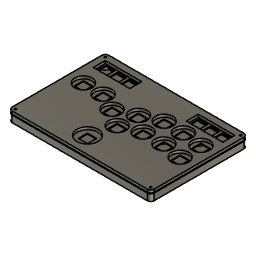
PitBox (Autodesk Fusion 360 design; units mm, degrees)
Autodesk Fusion 360 part; units mm, degrees
sketch "Sketch2" plane through (0, 0, 0) normal (0, 0, 1) x (1, 0, 0)
  circle A0 centre (22.2936, -55.3178) radius 12.0327
  circle A1 centre (51.9241, -55.2175) radius 12.0327
  circle A2 centre (78.346, -68.2028) radius 12.0327
  circle A3 centre (106.2419, -56.2403) radius 12.0327
  circle A4 centre (133.2453, -44.4382) radius 12.0327
  circle A5 centre (162.9862, -45.1702) radius 12.0327
  circle A6 centre (192.5566, -48.2686) radius 12.0327
  circle A7 centre (103.5847, -85.6403) radius 12.0327
  circle A8 centre (131.5808, -74.52) radius 12.0327
  circle A9 centre (162.7756, -74.3195) radius 12.0327
  circle A10 centre (192.2758, -79.3532) radius 12.0327
  circle A11 centre (93.8883, -120.7958) radius 15.0409
  line L0 (15.3935, -48.4178) -> (29.1935, -48.4178)
  line L1 (29.1935, -48.4178) -> (29.1935, -62.2178)
  line L2 (29.1935, -62.2178) -> (15.3935, -62.2178)
  line L3 (15.3935, -62.2178) -> (15.3935, -48.4178)
  line L4 (45.0241, -48.3175) -> (58.8241, -48.3175)
  line L5 (58.8241, -48.3175) -> (58.8241, -62.1175)
  line L6 (58.8241, -62.1175) -> (45.0241, -62.1175)
  line L7 (45.0241, -62.1175) -> (45.0241, -48.3175)
  line L8 (71.446, -61.3028) -> (85.246, -61.3028)
  line L9 (85.246, -61.3028) -> (85.246, -75.1028)
  line L10 (85.246, -75.1028) -> (71.446, -75.1028)
  line L11 (71.446, -75.1028) -> (71.446, -61.3028)
  line L12 (99.3419, -49.3403) -> (113.1419, -49.3403)
  line L13 (113.1419, -49.3403) -> (113.1419, -63.1403)
  line L14 (113.1419, -63.1403) -> (99.3419, -63.1403)
  line L15 (99.3419, -63.1403) -> (99.3419, -49.3403)
  line L16 (126.3453, -37.5382) -> (140.1453, -37.5382)
  line L17 (140.1453, -37.5382) -> (140.1453, -51.3382)
  line L18 (140.1453, -51.3382) -> (126.3453, -51.3382)
  line L19 (126.3453, -51.3382) -> (126.3453, -37.5382)
  line L20 (156.0862, -38.2702) -> (169.8862, -38.2702)
  line L21 (169.8862, -38.2702) -> (169.8862, -52.0702)
  line L22 (169.8862, -52.0702) -> (156.0862, -52.0702)
  line L23 (156.0862, -52.0702) -> (156.0862, -38.2702)
  line L24 (185.6566, -41.3686) -> (199.4566, -41.3686)
  line L25 (199.4566, -41.3686) -> (199.4566, -55.1686)
  line L26 (199.4566, -55.1686) -> (185.6566, -55.1686)
  line L27 (185.6566, -55.1686) -> (185.6566, -41.3686)
  line L28 (185.3758, -72.4532) -> (199.1758, -72.4532)
  line L29 (199.1758, -72.4532) -> (199.1758, -86.2532)
  line L30 (199.1758, -86.2532) -> (185.3758, -86.2532)
  line L31 (185.3758, -86.2532) -> (185.3758, -72.4532)
  line L32 (155.8756, -67.4195) -> (169.6756, -67.4195)
  line L33 (169.6756, -67.4195) -> (169.6756, -81.2195)
  line L34 (169.6756, -81.2195) -> (155.8756, -81.2195)
  line L35 (155.8756, -81.2195) -> (155.8756, -67.4195)
  line L36 (124.6808, -67.62) -> (138.4808, -67.62)
  line L37 (138.4808, -67.62) -> (138.4808, -81.42)
  line L38 (138.4808, -81.42) -> (124.6808, -81.42)
  line L39 (124.6808, -81.42) -> (124.6808, -67.62)
  line L40 (96.6847, -78.7403) -> (110.4846, -78.7403)
  line L41 (110.4846, -78.7403) -> (110.4846, -92.5403)
  line L42 (110.4846, -92.5403) -> (96.6847, -92.5403)
  line L43 (96.6847, -92.5403) -> (96.6847, -78.7403)
  line L44 (86.9883, -113.8959) -> (100.7883, -113.8959)
  line L45 (100.7883, -113.8959) -> (100.7883, -127.6959)
  line L46 (100.7883, -127.6959) -> (86.9883, -127.6959)
  line L47 (86.9883, -127.6959) -> (86.9883, -113.8959)
  line L48 (12.2471, -11.7471) -> (26.0471, -11.7471)
  line L49 (26.0471, -11.7471) -> (26.0471, -25.5471)
  line L50 (26.0471, -25.5471) -> (12.2471, -25.5471)
  line L51 (12.2471, -25.5471) -> (12.2471, -11.7471)
  line L52 (30.2471, -11.7471) -> (44.0471, -11.7471)
  line L53 (44.0471, -11.7471) -> (44.0471, -25.5471)
  line L54 (44.0471, -25.5471) -> (30.2471, -25.5471)
  line L55 (30.2471, -25.5471) -> (30.2471, -11.7471)
  line L56 (48.2471, -11.7471) -> (62.0471, -11.7471)
  line L57 (62.0471, -11.7471) -> (62.0471, -25.5471)
  line L58 (62.0471, -25.5471) -> (48.2471, -25.5471)
  line L59 (48.2471, -25.5471) -> (48.2471, -11.7471)
  line L60 (152.5223, -11.7471) -> (166.3223, -11.7471)
  line L61 (166.3223, -11.7471) -> (166.3223, -25.5471)
  line L62 (166.3223, -25.5471) -> (152.5223, -25.5471)
  line L63 (152.5223, -25.5471) -> (152.5223, -11.7471)
  line L64 (170.5223, -11.7471) -> (184.3223, -11.7471)
  line L65 (184.3223, -11.7471) -> (184.3223, -25.5471)
  line L66 (184.3223, -25.5471) -> (170.5223, -25.5471)
  line L67 (170.5223, -25.5471) -> (170.5223, -11.7471)
  line L68 (188.5223, -11.7471) -> (202.3223, -11.7471)
  line L69 (202.3223, -11.7471) -> (202.3223, -25.5471)
  line L70 (202.3223, -25.5471) -> (188.5223, -25.5471)
  line L71 (188.5223, -25.5471) -> (188.5223, -11.7471)
  line L72 (67.846, -4.145) -> (88.846, -4.145)
  line L73 (88.846, -4.145) -> (88.846, -55.145)
  line L74 (88.846, -55.145) -> (67.846, -55.145)
  line L75 (67.846, -55.145) -> (67.846, -4.145)
  line L76 (74.346, -2.845) -> (82.346, -2.845)
  line L77 (82.346, -2.845) -> (82.346, -4.145)
  line L78 (82.346, -4.145) -> (74.346, -4.145)
  line L79 (74.346, -4.145) -> (74.346, -2.845)
  circle A12 centre (72.646, -52.745) radius 1.25
  circle A13 centre (83.9813, -52.745) radius 1.25
  circle A14 centre (84.046, -6.145) radius 1.25
  circle A15 centre (72.646, -6.145) radius 1.25
  line L80 (0.0725, -0.0725) -> (214.4223, -0.0725)
  line L81 (214.4223, -0.0725) -> (214.4223, -145.9094)
  line L82 (214.4223, -145.9094) -> (0.0725, -145.9094)
  line L83 (0.0725, -145.9094) -> (0.0725, -0.0725)
  line L84 (10.1471, -10.1471) -> (64.1471, -10.1471)
  line L85 (64.1471, -10.1471) -> (64.1471, -27.1471)
  line L86 (64.1471, -27.1471) -> (10.1471, -27.1471)
  line L87 (10.1471, -27.1471) -> (10.1471, -10.1471)
  line L88 (150.4223, -10.1471) -> (204.4223, -10.1471)
  line L89 (204.4223, -10.1471) -> (204.4223, -27.1471)
  line L90 (204.4223, -27.1471) -> (150.4223, -27.1471)
  line L91 (150.4223, -27.1471) -> (150.4223, -10.1471)
  circle A16 centre (5.0725, -5.0725) radius 1.5
  circle A17 centre (209.4223, -5.0725) radius 1.5
  circle A18 centre (5.0725, -140.9094) radius 1.5
  circle A19 centre (209.4223, -140.9094) radius 1.5
  circle A20 centre (22.2936, -55.3178) radius 13.0327
  circle A21 centre (51.9241, -55.2175) radius 13.0327
  circle A22 centre (78.346, -68.2028) radius 13.0327
  circle A23 centre (106.2419, -56.2403) radius 13.0327
  circle A24 centre (133.2453, -44.4382) radius 13.0327
  circle A25 centre (162.9862, -45.1702) radius 13.0327
  circle A26 centre (192.5566, -48.2686) radius 13.0327
  circle A27 centre (103.5847, -85.6403) radius 13.0327
  circle A28 centre (131.5808, -74.52) radius 13.0327
  circle A29 centre (162.7756, -74.3195) radius 13.0327
  circle A30 centre (192.2758, -79.3532) radius 13.0327
  circle A31 centre (93.8883, -120.7958) radius 16.0409
  circle A32 centre (72.646, -6.145) radius 1
  circle A33 centre (84.046, -6.145) radius 1
  circle A34 centre (72.646, -6.145) radius 2
  circle A35 centre (84.046, -6.145) radius 2
  circle A36 centre (72.646, -52.745) radius 1
  circle A37 centre (83.9813, -52.745) radius 1
  circle A38 centre (72.646, -52.745) radius 2
  circle A39 centre (83.9813, -52.745) radius 2
  line L92 (72.646, -6.145) -> (84.046, -6.145)
  line L93 (84.846, 0.355) -> (71.846, 0.355)
  line L94 (71.846, 0.355) -> (71.846, -12.645)
  line L95 (71.846, -12.645) -> (84.846, -12.645)
  line L96 (84.846, -12.645) -> (84.846, 0.355)
  line L97 (84.846, 0.355) -> (71.846, -12.645) construction
  line L98 (71.846, 0.355) -> (84.846, -12.645) construction
  point P0 (34.3263, -55.3178)
  point P1 (63.9569, -55.2175)
  point P2 (90.3787, -68.2028)
  point P3 (118.2746, -56.2403)
  point P4 (145.2781, -44.4382)
  point P5 (175.019, -45.1702)
  point P6 (204.5894, -48.2686)
  point P7 (115.6174, -85.6403)
  point P8 (143.6135, -74.52)
  point P9 (174.8084, -74.3195)
  point P10 (204.3086, -79.3532)
  point P11 (108.9292, -120.7958)
  point P12 (73.896, -52.745)
  point P13 (85.2313, -52.745)
  point P14 (85.296, -6.145)
  point P15 (73.896, -6.145)
  point P16 (78.346, -6.145)
  dimension "d36" = 3
  dimension "d37" = 3
  dimension "d38" = 3
  dimension "d39" = 3
  dimension "d40" = 5
  dimension "d41" = 5
  dimension "d42" = 5
  dimension "d43" = 5
  dimension "d44" = 5
  dimension "d45" = 5
  dimension "d46" = 5
  dimension "d47" = 5
  dimension "d48" = -1
  dimension "d49" = -1
  dimension "d50" = -1
  dimension "d51" = -1
  dimension "d52" = -1
  dimension "d53" = -1
  dimension "d54" = -1
  dimension "d55" = -1
  dimension "d56" = -1
  dimension "d57" = -1
  dimension "d58" = -1
  dimension "d59" = -1
  dimension "d64" = 2
  dimension "d65" = 2
  dimension "d66" = 4
  dimension "d67" = 4
  dimension "d68" = 2
  dimension "d69" = 2
  dimension "d70" = 4
  dimension "d71" = 4
  dimension "d85" = 13
  dimension "d86" = 13
  constraint concentric A15 A32
  constraint concentric A14 A33
  constraint concentric A15 A34
  constraint concentric A33 A35
  constraint concentric A12 A36
  constraint concentric A13 A37
  constraint concentric A12 A38
  constraint concentric A37 A39
  constraint coincident A15.centre A32.centre
  constraint coincident A14.centre A33.centre
  constraint horizontal L93
  constraint perpendicular L93 L94
  constraint parallel L93 L95
  constraint parallel L94 L96
  constraint coincident L97 P16
  constraint coincident L98 P16
  constraint midpoint L92 P16
  measures "d36" diameter of A16
  measures "d37" diameter of A17
  measures "d38" diameter of A18
  measures "d39" diameter of A19
  measures "d40" distance of L80 A16.centre
  measures "d41" distance of L83 A16.centre
  measures "d42" distance of L80 A17.centre
  measures "d43" distance of L81 A17.centre
  measures "d44" distance of L81 A19.centre
  measures "d45" distance of L82 A19.centre
  measures "d46" distance of L82 A18.centre
  measures "d47" distance of L83 A18.centre
  measures "d64" diameter of A32
  measures "d65" diameter of A33
  measures "d66" diameter of A34
  measures "d67" diameter of A35
  measures "d68" diameter of A36
  measures "d69" diameter of A37
  measures "d70" diameter of A38
  measures "d71" diameter of A39
  measures "d85" distance of L94.end L95.end
  measures "d86" distance of L93.end L94.end
extrude "Extrude1" add sketch "Sketch2" along normal blind 4 contours L72 L76 L77 L78 L79 | L72 L78 A34 A35 L92 | L72 L76 L77 L79 L80 L94 L96 | L72 A34 L94 | A15 A34 L92 L94 | L72 A35 L96 | A14 A35 L92 L96 | L72 L73 L74 L75 A34 A35 L94 L95 L96 | L72 L73 L74 L75 L80 L81 L82 L83 L94 L96 | A34 A35 L92 L94 L95 L96 | A15 A34 L92 L94 | A15 A34 L94 | A14 A35 L96 | A14 A35 L92 L96 | A15 A32 L92 L94 | A15 A32 L92 L94 | A15 A32 L94 | A14 A33 L92 L96 | A14 A33 L96 | A14 A33 L92 L96 | A32 L94 | A32 L94 | A33 L96 | A33 L96 | A12 | A13 | A36 | A37 | A38 | A39 makes body 1
extrude "Extrude2" add sketch "Sketch2" against normal blind 1.2 separate body contours A0 | A1 | A2 | A3 | A4 | A5 | A6 | A7 | A8 | A9 | A10 | A11 | L72 L78 A34 A35 L92 | L72 A34 L94 | A15 A34 L92 L94 | L72 A35 L96 | A14 A35 L92 L96 | L72 L73 L74 L75 A34 A35 L94 L95 L96 | L72 L73 L74 L75 L80 L81 L82 L83 L94 L96 | A34 A35 L92 L94 L95 L96 | A15 A34 L92 L94 | A15 A34 L94 | A14 A35 L96 | A14 A35 L92 L96 | A15 A32 L92 L94 | A15 A32 L92 L94 | A15 A32 L94 | A14 A33 L92 L96 | A14 A33 L96 | A14 A33 L92 L96 | A32 L94 | A32 L94 | A33 L96 | A33 L96 | A12 | A13 | L84 L85 L86 L87 | L88 L89 L90 L91 | A20 | A21 | A22 | A23 | A24 | A25 | A26 | A27 | A28 | A29 | A30 | A31 | A36 | A37 | A38 | A39 makes body 2
extrude "Extrude3" add sketch "Sketch2" against normal blind 3.2 contours A15 A34 L92 L94 | A14 A35 L92 L96 | A15 A34 L92 L94 | A15 A34 L94 | A14 A35 L96 | A14 A35 L92 L96 | A15 A32 L92 L94 | A15 A32 L92 L94 | A15 A32 L94 | A14 A33 L92 L96 | A14 A33 L96 | A14 A33 L92 L96 | A12 | A13 | A38 | A39 bodies 2
extrude "Extrude4" cut 4 faces at (84.3645, -6.2433, -1.2) (72.9645, -6.2433, -1.2) (83.7735, -53.2021, -1.2) (72.4382, -53.2021, -1.2) along direction (0, 0, 1) blind 2 on bodies 2 bodies 2
sketch "Sketch3" plane through (0, 0, -1.2) normal (0, 0, -1) x (1, 0, 0)
  circle A0 centre (72.646, 6.145) radius 2
  circle A1 centre (84.046, 6.145) radius 2
  line L0 (48.2471, 25.5471) -> (62.0471, 25.5471)
  line L1 (62.0471, 25.5471) -> (62.0471, 11.7471)
  line L2 (62.0471, 11.7471) -> (48.2471, 11.7471)
  line L3 (48.2471, 11.7471) -> (48.2471, 25.5471)
  line L4 (86.9883, 127.6959) -> (100.7883, 127.6959)
  line L5 (100.7883, 127.6959) -> (100.7883, 113.8959)
  line L6 (100.7883, 113.8959) -> (86.9883, 113.8959)
  line L7 (86.9883, 113.8959) -> (86.9883, 127.6959)
  line L8 (188.5223, 25.5471) -> (202.3223, 25.5471)
  line L9 (202.3223, 25.5471) -> (202.3223, 11.7471)
  line L10 (202.3223, 11.7471) -> (188.5223, 11.7471)
  line L11 (188.5223, 11.7471) -> (188.5223, 25.5471)
  line L12 (30.2471, 25.5471) -> (44.0471, 25.5471)
  line L13 (44.0471, 25.5471) -> (44.0471, 11.7471)
  line L14 (44.0471, 11.7471) -> (30.2471, 11.7471)
  line L15 (30.2471, 11.7471) -> (30.2471, 25.5471)
  line L16 (156.0862, 52.0702) -> (169.8862, 52.0702)
  line L17 (169.8862, 52.0702) -> (169.8862, 38.2702)
  line L18 (169.8862, 38.2702) -> (156.0862, 38.2702)
  line L19 (156.0862, 38.2702) -> (156.0862, 52.0702)
  circle A2 centre (209.4223, 140.9094) radius 1.5
  line L20 (170.5223, 25.5471) -> (184.3223, 25.5471)
  line L21 (184.3223, 25.5471) -> (184.3223, 11.7471)
  line L22 (184.3223, 11.7471) -> (170.5223, 11.7471)
  line L23 (170.5223, 11.7471) -> (170.5223, 25.5471)
  line L24 (71.446, 75.1028) -> (85.246, 75.1028)
  line L25 (85.246, 75.1028) -> (85.246, 61.3028)
  line L26 (85.246, 61.3028) -> (71.446, 61.3028)
  line L27 (71.446, 61.3028) -> (71.446, 75.1028)
  line L28 (96.6847, 92.5403) -> (110.4846, 92.5403)
  line L29 (110.4846, 92.5403) -> (110.4846, 78.7403)
  line L30 (110.4846, 78.7403) -> (96.6847, 78.7403)
  line L31 (96.6847, 78.7403) -> (96.6847, 92.5403)
  circle A3 centre (5.0725, 140.9094) radius 1.5
  line L32 (185.3758, 86.2532) -> (199.1758, 86.2532)
  line L33 (199.1758, 86.2532) -> (199.1758, 72.4532)
  line L34 (199.1758, 72.4532) -> (185.3758, 72.4532)
  line L35 (185.3758, 72.4532) -> (185.3758, 86.2532)
  line L36 (15.3935, 62.2178) -> (29.1935, 62.2178)
  line L37 (29.1935, 62.2178) -> (29.1935, 48.4178)
  line L38 (29.1935, 48.4178) -> (15.3935, 48.4178)
  line L39 (15.3935, 48.4178) -> (15.3935, 62.2178)
  line L40 (152.5223, 25.5471) -> (166.3223, 25.5471)
  line L41 (166.3223, 25.5471) -> (166.3223, 11.7471)
  line L42 (166.3223, 11.7471) -> (152.5223, 11.7471)
  line L43 (152.5223, 11.7471) -> (152.5223, 25.5471)
  line L44 (12.2471, 25.5471) -> (26.0471, 25.5471)
  line L45 (26.0471, 25.5471) -> (26.0471, 11.7471)
  line L46 (26.0471, 11.7471) -> (12.2471, 11.7471)
  line L47 (12.2471, 11.7471) -> (12.2471, 25.5471)
  line L48 (155.8756, 81.2195) -> (169.6756, 81.2195)
  line L49 (169.6756, 81.2195) -> (169.6756, 67.4195)
  line L50 (169.6756, 67.4195) -> (155.8756, 67.4195)
  line L51 (155.8756, 67.4195) -> (155.8756, 81.2195)
  line L52 (126.3453, 51.3382) -> (140.1453, 51.3382)
  line L53 (140.1453, 51.3382) -> (140.1453, 37.5382)
  line L54 (140.1453, 37.5382) -> (126.3453, 37.5382)
  line L55 (126.3453, 37.5382) -> (126.3453, 51.3382)
  line L56 (185.6566, 55.1686) -> (199.4566, 55.1686)
  line L57 (199.4566, 55.1686) -> (199.4566, 41.3686)
  line L58 (199.4566, 41.3686) -> (185.6566, 41.3686)
  line L59 (185.6566, 41.3686) -> (185.6566, 55.1686)
  line L60 (99.3419, 63.1403) -> (113.1419, 63.1403)
  line L61 (113.1419, 63.1403) -> (113.1419, 49.3403)
  line L62 (113.1419, 49.3403) -> (99.3419, 49.3403)
  line L63 (99.3419, 49.3403) -> (99.3419, 63.1403)
  circle A4 centre (209.4223, 5.0725) radius 1.5
  line L64 (45.0241, 62.1175) -> (58.8241, 62.1175)
  line L65 (58.8241, 62.1175) -> (58.8241, 48.3175)
  line L66 (58.8241, 48.3175) -> (45.0241, 48.3175)
  line L67 (45.0241, 48.3175) -> (45.0241, 62.1175)
  line L68 (124.6808, 81.42) -> (138.4808, 81.42)
  line L69 (138.4808, 81.42) -> (138.4808, 67.62)
  line L70 (138.4808, 67.62) -> (124.6808, 67.62)
  line L71 (124.6808, 67.62) -> (124.6808, 81.42)
  circle A5 centre (5.0725, 5.0725) radius 1.5
  line L72 (214.4223, 145.9094) -> (0.0725, 145.9094)
  line L73 (0.0725, 145.9094) -> (0.0725, 0.0725)
  line L74 (84.846, 0.0725) -> (214.4223, 0.0725)
  line L75 (214.4223, 0.0725) -> (214.4223, 145.9094)
  circle A6 centre (72.646, 52.745) radius 2
  circle A7 centre (83.9813, 52.745) radius 2
  line L76 (152.5223, 25.5471) -> (166.3223, 25.5471)
  line L77 (188.5223, 25.5471) -> (202.3223, 25.5471)
  line L78 (170.5223, 11.7471) -> (170.5223, 25.5471)
  line L79 (45.0241, 62.1175) -> (58.8241, 62.1175)
  line L80 (184.3223, 11.7471) -> (170.5223, 11.7471)
  line L81 (169.8862, 38.2702) -> (156.0862, 38.2702)
  line L82 (184.3223, 25.5471) -> (184.3223, 11.7471)
  line L83 (156.0862, 38.2702) -> (156.0862, 52.0702)
  line L84 (45.0241, 48.3175) -> (45.0241, 62.1175)
  line L85 (71.446, 61.3028) -> (71.446, 75.1028)
  line L86 (86.9883, 113.8959) -> (86.9883, 127.6959)
  line L87 (126.3453, 37.5382) -> (126.3453, 51.3382)
  line L88 (124.6808, 81.42) -> (138.4808, 81.42)
  line L89 (0.0725, 145.9094) -> (0.0725, 0.0725)
  line L90 (138.4808, 67.62) -> (124.6808, 67.62)
  line L91 (214.4223, 145.9094) -> (0.0725, 145.9094)
  line L92 (0.0725, 0.0725) -> (214.4223, 0.0725)
  line L93 (214.4223, 0.0725) -> (214.4223, 145.9094)
  line L94 (86.9883, 127.6959) -> (100.7883, 127.6959)
  line L95 (110.4846, 92.5403) -> (110.4846, 78.7403)
  line L96 (124.6808, 67.62) -> (124.6808, 81.42)
  line L97 (85.246, 75.1028) -> (85.246, 61.3028)
  line L98 (85.246, 61.3028) -> (71.446, 61.3028)
  line L99 (71.446, 75.1028) -> (85.246, 75.1028)
  line L100 (113.1419, 63.1403) -> (113.1419, 49.3403)
  line L101 (199.1758, 86.2532) -> (199.1758, 72.4532)
  line L102 (100.7883, 113.8959) -> (86.9883, 113.8959)
  line L103 (138.4808, 81.42) -> (138.4808, 67.62)
  line L104 (100.7883, 127.6959) -> (100.7883, 113.8959)
  line L105 (185.3758, 86.2532) -> (199.1758, 86.2532)
  line L106 (96.6847, 92.5403) -> (110.4846, 92.5403)
  line L107 (199.1758, 72.4532) -> (185.3758, 72.4532)
  line L108 (185.3758, 72.4532) -> (185.3758, 86.2532)
  line L109 (140.1453, 37.5382) -> (126.3453, 37.5382)
  line L110 (110.4846, 78.7403) -> (96.6847, 78.7403)
  line L111 (155.8756, 81.2195) -> (169.6756, 81.2195)
  line L112 (156.0862, 52.0702) -> (169.8862, 52.0702)
  line L113 (15.3935, 62.2178) -> (29.1935, 62.2178)
  line L114 (166.3223, 25.5471) -> (166.3223, 11.7471)
  line L115 (99.3419, 63.1403) -> (113.1419, 63.1403)
  line L116 (185.6566, 41.3686) -> (185.6566, 55.1686)
  line L117 (185.6566, 55.1686) -> (199.4566, 55.1686)
  line L118 (199.4566, 55.1686) -> (199.4566, 41.3686)
  line L119 (155.8756, 67.4195) -> (155.8756, 81.2195)
  line L120 (199.4566, 41.3686) -> (185.6566, 41.3686)
  line L121 (169.8862, 52.0702) -> (169.8862, 38.2702)
  line L122 (152.5223, 11.7471) -> (152.5223, 25.5471)
  line L123 (166.3223, 11.7471) -> (152.5223, 11.7471)
  line L124 (140.1453, 51.3382) -> (140.1453, 37.5382)
  line L125 (126.3453, 51.3382) -> (140.1453, 51.3382)
  circle A8 centre (209.4223, 140.9094) radius 1.5
  line L126 (169.6756, 81.2195) -> (169.6756, 67.4195)
  line L127 (169.6756, 67.4195) -> (155.8756, 67.4195)
  line L128 (96.6847, 78.7403) -> (96.6847, 92.5403)
  circle A9 centre (209.4223, 5.0725) radius 1.5
  line L129 (58.8241, 62.1175) -> (58.8241, 48.3175)
  circle A10 centre (5.0725, 140.9094) radius 1.5
  line L130 (15.3935, 48.4178) -> (15.3935, 62.2178)
  circle A11 centre (72.646, 52.745) radius 2
  line L131 (202.3223, 25.5471) -> (202.3223, 11.7471)
  line L132 (170.5223, 25.5471) -> (184.3223, 25.5471)
  line L133 (99.3419, 49.3403) -> (99.3419, 63.1403)
  line L134 (188.5223, 11.7471) -> (188.5223, 25.5471)
  line L135 (29.1935, 48.4178) -> (15.3935, 48.4178)
  circle A12 centre (83.9813, 52.745) radius 2
  line L136 (29.1935, 62.2178) -> (29.1935, 48.4178)
  line L137 (202.3223, 11.7471) -> (188.5223, 11.7471)
  line L138 (58.8241, 48.3175) -> (45.0241, 48.3175)
  line L139 (48.2471, 11.7471) -> (48.2471, 25.5471)
  line L140 (48.2471, 25.5471) -> (62.0471, 25.5471)
  circle A13 centre (84.046, 6.145) radius 2
  line L141 (44.0471, 25.5471) -> (44.0471, 11.7471)
  circle A14 centre (5.0725, 5.0725) radius 1.5
  line L142 (30.2471, 11.7471) -> (30.2471, 25.5471)
  line L143 (113.1419, 49.3403) -> (99.3419, 49.3403)
  circle A15 centre (72.646, 6.145) radius 2
  line L144 (62.0471, 25.5471) -> (62.0471, 11.7471)
  line L145 (62.0471, 11.7471) -> (48.2471, 11.7471)
  line L146 (44.0471, 11.7471) -> (30.2471, 11.7471)
  line L147 (12.2471, 11.7471) -> (12.2471, 25.5471)
  line L148 (30.2471, 25.5471) -> (44.0471, 25.5471)
  line L149 (12.2471, 25.5471) -> (26.0471, 25.5471)
  line L150 (26.0471, 11.7471) -> (12.2471, 11.7471)
  line L151 (26.0471, 25.5471) -> (26.0471, 11.7471)
  circle A16 centre (209.4223, 140.9094) radius 5
  circle A17 centre (5.0725, 140.9094) radius 5
  circle A18 centre (5.0725, 5.0725) radius 5
  circle A19 centre (209.4223, 5.0725) radius 5
  line L152 (209.4223, 5.0725) -> (5.0725, 5.0725)
  line L153 (5.0725, 5.0725) -> (5.0725, 140.9094)
  line L154 (5.0725, 140.9094) -> (209.4223, 140.9094)
  line L155 (209.4223, 140.9094) -> (209.4223, 5.0725)
  line L156 (93, 2) -> (64, 2)
  line L157 (64, 2) -> (64, 6)
  line L158 (64, 6) -> (93, 6)
  line L159 (93, 6) -> (93, 2)
  line L160 (71.846, 4.145) -> (72.646, 4.145)
  line L161 (72.646, 4.145) -> (84.046, 4.145)
  line L162 (84.046, 4.145) -> (84.846, 4.145)
  line L163 (84.846, 4.145) -> (84.846, 0.0725)
  line L164 (0.0725, 0.0725) -> (71.846, 0.0725)
  line L165 (71.846, 0.0725) -> (71.846, 4.145)
  line L166 (72.646, 6.145) -> (84.046, 6.145)
  line L167 (84.846, -0.355) -> (71.846, -0.355)
  line L168 (71.846, -0.355) -> (71.846, 12.645)
  line L169 (71.846, 12.645) -> (84.846, 12.645)
  line L170 (84.846, 12.645) -> (84.846, -0.355)
  line L171 (84.846, -0.355) -> (71.846, 12.645) construction
  line L172 (71.846, -0.355) -> (84.846, 12.645) construction
  circle A20 centre (104, 71) radius 3
  circle A21 centre (144.0162, 91.8271) radius 3
  circle A22 centre (176, 92) radius 3
  circle A23 centre (37, 37) radius 3
  circle A24 centre (37, 72) radius 3
  circle A25 centre (84, 99) radius 3
  circle A26 centre (115, 109) radius 3
  circle A27 centre (142, 18) radius 3
  circle A28 centre (177.3097, 34.7488) radius 3
  circle A29 centre (147, 60) radius 3
  circle A30 centre (62, 80) radius 3
  point P0 (78.5, 6)
  point P1 (78.346, 6.145)
  dimension "d76" = 10
  dimension "d77" = 10
  dimension "d78" = 10
  dimension "d79" = 10
  dimension "d87" = 13
  dimension "d88" = 13
  constraint concentric A8 A16
  constraint concentric A3 A17
  constraint concentric A5 A18
  constraint concentric A4 A19
  constraint horizontal L152
  constraint vertical L153
  constraint horizontal L154
  constraint vertical L155
  constraint coincident A3.centre A10.centre
  constraint coincident A4.centre A9.centre
  constraint horizontal L156
  constraint vertical L157
  constraint horizontal L158
  constraint vertical L159
  constraint midpoint L158 P0
  constraint coincident A0.centre A15.centre
  constraint coincident A1.centre A13.centre
  constraint parallel L158 L166
  constraint horizontal L167
  constraint perpendicular L167 L168
  constraint parallel L167 L169
  constraint parallel L168 L170
  constraint coincident L171 P1
  constraint coincident L172 P1
  constraint midpoint L166 P1
  measures "d76" diameter of A16
  measures "d77" diameter of A17
  measures "d78" diameter of A18
  measures "d79" diameter of A19
  measures "d87" distance of L168.end L169.end
  measures "d88" distance of L167.end L168.end
extrude "Extrude5" add sketch "Sketch3" along normal blind 8.5 separate body contours L92 A18 L152 L156 L157 L164 L165 L168 | A5 A14 A18 L152 L153 | A5 A14 A18 L152 L153 | L73 L89 A17 A18 L153 | L73 L89 L92 A18 L164 | L74 L92 A19 L152 L156 L159 L163 L170 | A3 A10 A17 L153 L154 | A3 A10 A17 L153 L154 | A4 A9 A19 L152 L155 | A4 A9 A19 L152 L155 | L72 L73 L89 L91 A17 | L72 L91 A16 A17 L154 | L74 L75 L92 L93 A19 | L75 L93 A16 A19 L155 | A2 A8 A16 L154 L155 | A2 A8 A16 L154 L155 | L72 L75 L91 L93 A16 makes body 3
sketch "Sketch5" plane through (0, 0, -9.7) normal (0, 0, -1) x (1, 0, 0)
  circle A0 centre (209.4223, 140.9094) radius 1.5
  circle A1 centre (209.4223, 5.0725) radius 1.5
  circle A2 centre (5.0725, 5.0725) radius 1.5
  circle A3 centre (5.0725, 140.9094) radius 1.5
  line L0 (214.4223, 0.0725) -> (214.4223, 145.9094)
  line L1 (214.4223, 145.9094) -> (0.0725, 145.9094)
  line L2 (0.0725, 145.9094) -> (0.0725, 0.0725)
  line L3 (84.846, 0.0725) -> (214.4223, 0.0725)
  line L4 (214.4223, 0.0725) -> (0.0725, 0.0725)
  line L5 (0.0725, 0.0725) -> (0.0725, 145.9094)
  line L6 (0.0725, 145.9094) -> (214.4223, 145.9094)
  line L7 (214.4223, 145.9094) -> (214.4223, 0.0725)
  circle A4 centre (209.4223, 5.0725) radius 1.5
  circle A5 centre (5.0725, 5.0725) radius 1.5
  circle A6 centre (209.4223, 140.9094) radius 1.5
  circle A7 centre (5.0725, 140.9094) radius 1.5
  line L8 (93, 2) -> (84.846, 2)
  line L9 (84.846, 2) -> (84.846, 0.0725)
  line L10 (0.0725, 0.0725) -> (71.846, 0.0725)
  line L11 (71.846, 0.0725) -> (71.846, 2)
  line L12 (71.846, 2) -> (64, 2)
  line L13 (64, 2) -> (64, 5.0725)
  line L14 (64, 5.0725) -> (10.0725, 5.0725)
  arc A8 (10.0725, 5.0725) -> (5.0725, 10.0725) centre (5.0725, 5.0725) ccw
  line L15 (5.0725, 10.0725) -> (5.0725, 135.9094)
  arc A9 (5.0725, 135.9094) -> (10.0725, 140.9094) centre (5.0725, 140.9094) ccw
  line L16 (10.0725, 140.9094) -> (204.4223, 140.9094)
  arc A10 (204.4223, 140.9094) -> (209.4223, 135.9094) centre (209.4223, 140.9094) ccw
  line L17 (209.4223, 135.9094) -> (209.4223, 10.0725)
  arc A11 (209.4223, 10.0725) -> (204.4223, 5.0725) centre (209.4223, 5.0725) ccw
  line L18 (204.4223, 5.0725) -> (93, 5.0725)
  line L19 (93, 5.0725) -> (93, 2)
  constraint horizontal L4
  constraint vertical L5
  constraint horizontal L6
  constraint vertical L7
  constraint coincident L1.end L2.start
  constraint coincident L0.start L3.end
  constraint concentric A1 A4
  constraint concentric A0 A6
extrude "Extrude6" add sketch "Sketch5" along normal blind 1.5 contours A0 A6 | A1 A4 | A2 A5 | A3 A7 | L0 L1 L2 L3 L4 L5 L6 L7 L8 L9 L10 L11 L12 L13 L14 A8 L15 A9 L16 A10 L17 A11 L18 L19 | L4 L8 L9 L11 L12 L13 L14 A8 L15 A9 L16 A10 L17 A11 L18 L19 bodies 3
fillet "Fillet1" radius 5 12 edges at (0.0725, -145.9094, 2) (0.0725, -0.0725, 2) (214.4223, -0.0725, 2) (214.4223, -145.9094, 2) (0.0725, -145.9094, -0.6) (0.0725, -0.0725, -0.6) (214.4223, -0.0725, -0.6) (214.4223, -145.9094, -0.6) (0.0725, -145.9094, -6.2) (0.0725, -0.0725, -6.2) (214.4223, -0.0725, -6.2) (214.4223, -145.9094, -6.2) on bodies 1 2 3
extrude "Extrude12" add sketch "Sketch3" along normal blind 8.4 contours A20 | A21 | A22 | A23 | A24 | A25 | A26 | A27 | A28 | A29 | A30 bodies 2
move_face "OffsetFaces1" offset -0.5 8 faces at (186.4223, -27.1471, 1.3333) (46.1471, -27.1471, 2.6667) (10.1471, -21.4805, 1.3333) (64.1471, -15.8138, 1.3333) (28.1471, -10.1471, 1.3333) (168.4223, -10.1471, 1.3333) (204.4223, -15.8138, 1.3333) (150.4223, -21.4805, 1.3333) on bodies 1
named bodies: "Top Case", "Plate", "Bottom Case"
